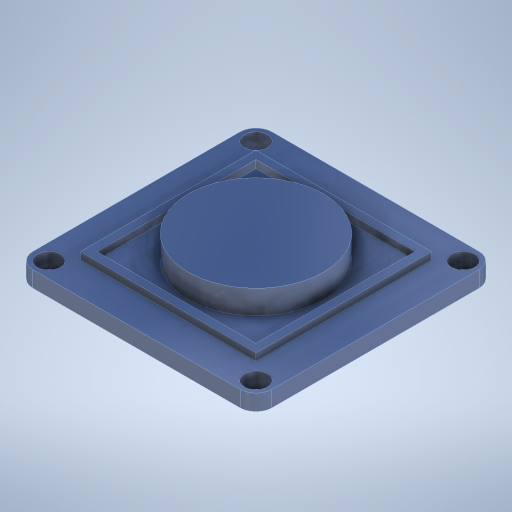
# Autodesk Inventor part: Tapa trasera
Saved by Autodesk Inventor 2023 (Build 270158000, 158)
## iProperties
Created: 2023-03-20
Part Number: Tapa trasera
Material: Plástico PET
Document SubType Name: Modeling
Designer: sergi
Density: 1.541 g/cm^3
Appearance: Satinado con motas - Azul
Author: sergi
Autodesk Inventor part; units mm, degrees
ref_plane "YZ Plane" through (0, 0, 0) normal (1, 0, 0) x (0, 1, 0)
ref_plane "XZ Plane" through (0, 0, 0) normal (0, 1, 0) x (-1, 0, 0)
ref_plane "XY Plane" through (0, 0, 0) normal (0, 0, 1) x (1, 0, 0)
sketch "Boceto1" plane through (0, 0, 0) normal (0, 1, 0) x (-1, 0, 0)
  line L0 (-13, 15) -> (13, 15)
  line L1 (15, 13) -> (15, -13)
  line L2 (13, -15) -> (-13, -15)
  line L3 (-15, -13) -> (-15, 13)
  line L4 (-15, 15) -> (15, -15) construction
  line L5 (15, 15) -> (-15, -15) construction
  arc A0 (13, -15) -> (15, -13) centre (13, -13) ccw
  arc A1 (15, 13) -> (13, 15) centre (13, 13) ccw
  arc A2 (-13, 15) -> (-15, 13) centre (-13, 13) ccw
  arc A3 (-15, -13) -> (-13, -15) centre (-13, -13) ccw
  point P0 (0, 0)
  dimension "d0" = 30
  dimension "d1" = 30
  dimension "d2" = 2
  constraints: 12 end point, 8 point on circle, 8 point on line, 8 tangent, 4 centre point, 3 equal radius, 2 midpoint, 2 parallel, 1 horizontal, 1 perpendicular
  measures "d0" distance of L4.end L5.end
  measures "d1" distance of L5.start L4.end
  measures "d2" radius of A0
extrude "Extrusión1" add sketch "Boceto1" along normal blind 2
sketch "Boceto2" plane through (0, 2, 0) normal (0, 1, 0) x (1, 0, 0)
  circle A0 centre (0, 0) radius 8.5
  dimension "d5" = 17
  constraints: 1 centre point, 1 coincident
  measures "d5" diameter of A0
extrude "Extrusión2" add sketch "Boceto2" along normal blind 3
sketch "Boceto3" plane through (0, 2, 0) normal (0, 1, 0) x (1, 0, 0)
  line L0 (10, -10) -> (-10, -10)
  line L1 (-10, -10) -> (-10, 10)
  line L2 (-10, 10) -> (10, 10)
  line L3 (10, 10) -> (10, -10)
  line L4 (10, -10) -> (-10, 10) construction
  line L5 (-10, -10) -> (10, 10) construction
  line L6 (11, -11) -> (-11, -11)
  line L7 (-11, -11) -> (-11, 11)
  line L8 (-11, 11) -> (11, 11)
  line L9 (11, 11) -> (11, -11)
  line L10 (11, -11) -> (-11, 11) construction
  line L11 (-11, -11) -> (11, 11) construction
  point P0 (0, 0)
  dimension "d8" = 1
  dimension "d9" = 1
  dimension "d10" = 10
  dimension "d11" = 10
  constraints: 24 end point, 4 midpoint, 4 parallel, 2 horizontal, 2 perpendicular
  measures "d8" distance between parallel lines of L7 L1
  measures "d9" distance between parallel lines of L0 L6
  measures "d10" distance from line of point (0, 0) L3
  measures "d11" distance from line of point (0, 0) L0
extrude "Extrusión3" add sketch "Boceto3" along normal blind 1
sketch "Boceto4" plane through (0, 0, 0) normal (0, -1, 0) x (1, 0, 0)
  point P0 (13, -13)
  point P1 (-13, -13)
hole "Agujero1" at (13, 0, -13) at (-13, 0, -13) direction (0, 1, 0) diameter 2.9 end through all
sketch "Boceto5" plane through (0, 0, 0) normal (0, -1, 0) x (1, 0, 0)
  point P0 (-13, 13)
hole "Agujero2" at (-13, 0, 13) direction (0, 1, 0) diameter 2.9 end through all
sketch "Boceto6" plane through (0, 0, 0) normal (0, -1, 0) x (1, 0, 0)
  point P0 (13, 13)
hole "Agujero3" at (13, 0, 13) direction (0, 1, 0) diameter 2.9 end through all
